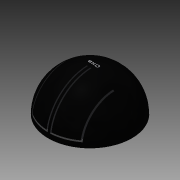
# Autodesk Inventor part: ORB-top
Saved by Autodesk Inventor 2015 (Build 190159000, 159)
## iProperties
Created: 2014-12-21
Part Number: ORB-top
Material: Generic
Document SubType Name: Modeling
Designer: Sudhar
Density: 1 g/cm^3
Appearance: Default
Author: Sudhar
Autodesk Inventor part; units mm, degrees
ref_plane "YZ Plane" through (0, 0, 0) normal (1, 0, 0) x (0, 1, 0)
sketch "Sketch1" plane through (0, 0, 0) normal (0, 0, 1) x (1, 0, 0)
  arc A0 (41.3405, 2.1184) -> (-3.1095, 46.5684) centre (-3.1095, 2.1184) ccw
  line L0 (-3.1095, 46.5684) -> (-3.1095, 2.1184)
  line L1 (41.3405, 2.1184) -> (-3.1095, 2.1184)
  dimension "d0" = 88.9
  constraints: 4 end point, 2 point on circle, 1 centre point, 1 perpendicular, 1 vertical
  measures "d0" diameter of A0
revolve "Revolution1" add sketch "Sketch1" angle 360 about axis through (-3.1095, 46.5684, 0) along (0, -1, 0)
shell "Shell1" thickness 3.175 removed faces 1 at (2.5499, 2.1184, 0)
ref_plane "Work Plane1" through (-3.1095, 2.1184, 44.45) normal (0, 0, 1) x (1, 0, 0)
sketch "Sketch2" plane through (-3.1095, 2.1184, 44.45) normal (0, 0, 1) x (1, 0, 0)
  line L0 (-26.3059, 36.8636) -> (-26.3059, 8.2886)
  line L1 (-23.1309, 5.1136) -> (-0.9059, 5.1136)
  line L2 (-0.9059, 5.1136) -> (-0.9059, 45.5389)
  line L3 (-0.9059, 45.5389) -> (1.6341, 45.5389)
  line L4 (1.6341, 45.5389) -> (1.6341, 5.1136)
  line L5 (1.6341, 5.1136) -> (27.0341, 5.1136)
  line L6 (27.0341, 5.1136) -> (27.0341, 36.8636)
  line L7 (-26.3059, 36.8636) -> (-25.0359, 36.8636)
  line L8 (-25.0359, 36.8636) -> (-25.0359, 9.7512)
  line L9 (-21.8609, 6.5762) -> (-2.1759, 6.5762)
  line L10 (-2.1759, 6.5762) -> (-2.1759, 46.5552)
  line L11 (-2.1759, 46.5552) -> (2.9041, 46.5552)
  line L12 (2.9041, 46.5552) -> (2.9041, 6.5762)
  line L13 (2.9041, 6.5762) -> (25.7641, 6.5762)
  line L14 (25.7641, 6.5762) -> (25.7641, 36.8636)
  line L15 (25.7641, 36.8636) -> (27.0341, 36.8636)
  arc A0 (-26.3059, 8.2886) -> (-23.1309, 5.1136) centre (-23.1309, 8.2886) ccw
  arc A1 (-25.0359, 9.7512) -> (-21.8609, 6.5762) centre (-21.8609, 9.7512) ccw
  point P0 (-26.3059, 5.1136)
  point P1 (-25.0359, 6.5762)
  dimension "d3" = 25.4
  dimension "d4" = 25.4
  dimension "d5" = 2.54
  dimension "d6" = 31.75
  dimension "d7" = 31.75
  dimension "d8" = 1.27
  dimension "d9" = 1.27
  dimension "d10" = 1.27
  dimension "d11" = 1.27
  dimension "d16" = 3.175
  constraints: 32 end point, 9 perpendicular, 9 point on line, 4 point on circle, 4 tangent, 2 centre point, 2 parallel, 1 equal radius, 1 horizontal, 1 vertical
  measures "d3" distance of point (-26.306, 5.114) L1.end
  measures "d4" distance of L4.end L5.end
  measures "d5" distance of L2.end L3.end
  measures "d6" distance of L0.start point (-26.306, 5.114)
  measures "d7" distance of L5.end L6.end
  measures "d8" distance of L0.start L7.end
  measures "d9" horizontal distance of L2.end L10.end
  measures "d10" horizontal distance of L3.end L11.end
  measures "d11" horizontal distance of L5.end L13.end
  measures "d16" radius of A0
extrude "Extrusion1" cut sketch "Sketch2" against normal blind 43.18
ref_plane "Work Plane2" through (-3.1095, 46.5684, 0) normal (0, 1, 0) x (-1, 0, 0)
sketch "Sketch3" plane through (-3.1095, 46.5684, 0) normal (0, 1, 0) x (-1, 0, 0)
  line L0 (-11.0824, -2.3342) -> (10.5197, -2.3342) construction
  line L1 (10.5197, -2.3342) -> (10.5197, -7.7787) construction
  line L2 (10.5197, -7.7787) -> (-11.0824, -7.7787) construction
  line L3 (-11.0824, -7.7787) -> (-11.0824, -2.3342) construction
  spline S0 degree 2 poles (-5.7235, -3.0556) (-5.7235, -2.6408) (-5.426, -2.3342) (-5.0081, -2.3342) knots 0 0 0 1 2 2 2
  line L4 (-5.0081, -2.3342) -> (-2.901, -2.3342)
  spline S1 degree 2 poles (-2.901, -2.3342) (-2.4892, -2.3342) (-2.1916, -2.6378) (-2.1916, -3.0556) knots 0 0 0 1 2 2 2
  line L5 (-2.1916, -3.0556) -> (-2.1916, -4.6607)
  spline S2 degree 2 poles (-2.1916, -4.6607) (-2.1916, -5.0816) (-2.4892, -5.3822) (-2.901, -5.3822) knots 0 0 0 1 2 2 2
  line L6 (-2.901, -5.3822) -> (-5.0081, -5.3822)
  spline S3 degree 2 poles (-5.0081, -5.3822) (-5.426, -5.3822) (-5.7235, -5.0756) (-5.7235, -4.6607) knots 0 0 0 1 2 2 2
  line L7 (-5.7235, -4.6607) -> (-5.7235, -3.0556)
  line L8 (-5.2155, -4.9583) -> (-2.6936, -4.9583)
  line L9 (-2.6936, -4.9583) -> (-2.6936, -2.749)
  line L10 (-2.6936, -2.749) -> (-5.2155, -2.749)
  line L11 (-5.2155, -2.749) -> (-5.2155, -4.9583)
  line L12 (-0.857, -5.3822) -> (-0.857, -2.8812)
  line L13 (-0.857, -2.8812) -> (1.157, -2.8812)
  spline S4 degree 2 poles (1.157, -2.8812) (1.4365, -2.8812) (1.68, -3.1097) (1.68, -3.3652) knots 0 0 0 1 2 2 2
  line L14 (1.68, -3.3652) -> (1.68, -3.9243)
  spline S5 degree 2 poles (1.68, -3.9243) (1.68, -4.1768) (1.4365, -4.4022) (1.157, -4.4022) knots 0 0 0 1 2 2 2
  line L15 (1.157, -4.4022) -> (0.8233, -4.4022)
  line L16 (0.8233, -4.4022) -> (1.9265, -5.3822)
  line L17 (1.9265, -5.3822) -> (1.2953, -5.3822)
  line L18 (1.2953, -5.3822) -> (0.2973, -4.4022)
  line L19 (0.2973, -4.4022) -> (-0.385, -4.4022)
  line L20 (-0.385, -4.4022) -> (-0.385, -5.3822)
  line L21 (-0.385, -5.3822) -> (-0.857, -5.3822)
  line L22 (0.9496, -3.248) -> (-0.385, -3.248)
  line L23 (-0.385, -3.248) -> (-0.385, -4.0535)
  line L24 (-0.385, -4.0535) -> (0.9496, -4.0535)
  spline S6 degree 2 poles (0.9496, -4.0535) (1.1089, -4.0535) (1.2171, -3.9513) (1.2171, -3.801) knots 0 0 0 1 2 2 2
  line L25 (1.2171, -3.801) -> (1.2171, -3.5005)
  spline S7 degree 2 poles (1.2171, -3.5005) (1.2171, -3.3622) (1.1029, -3.248) (0.9496, -3.248) knots 0 0 0 1 2 2 2
  line L26 (2.7592, -5.3822) -> (2.7592, -2.8812)
  line L27 (2.7592, -2.8812) -> (4.8723, -2.8812)
  spline S8 degree 2 poles (4.8723, -2.8812) (5.1609, -2.8812) (5.4194, -3.1157) (5.4194, -3.3712) knots 0 0 0 1 2 2 2
  line L28 (5.4194, -3.3712) -> (5.4194, -3.6598)
  spline S9 degree 2 poles (5.4194, -3.6598) (5.4194, -3.8582) (5.212, -4.0626) (4.9865, -4.0866) knots 0 0 0 1 2 2 2
  spline S10 degree 2 poles (4.9865, -4.0866) (5.206, -4.1107) (5.4374, -4.3601) (5.4374, -4.5706) knots 0 0 0 1 2 2 2
  line L29 (5.4374, -4.5706) -> (5.4374, -4.8922)
  spline S11 degree 2 poles (5.4374, -4.8922) (5.4374, -5.1387) (5.0797, -5.3822) (4.713, -5.3822) knots 0 0 0 1 2 2 2
  line L30 (4.713, -5.3822) -> (2.7592, -5.3822)
  line L31 (3.2311, -4.2549) -> (3.2311, -5.0154)
  line L32 (3.2311, -5.0154) -> (4.6829, -5.0154)
  spline S12 degree 2 poles (4.6829, -5.0154) (4.8453, -5.0154) (4.9685, -4.8922) (4.9685, -4.7329) knots 0 0 0 1 2 2 2
  line L33 (4.9685, -4.7329) -> (4.9685, -4.5375)
  spline S13 degree 2 poles (4.9685, -4.5375) (4.9685, -4.3812) (4.8423, -4.2549) (4.6829, -4.2549) knots 0 0 0 1 2 2 2
  line L34 (4.6829, -4.2549) -> (3.2311, -4.2549)
  line L35 (4.9505, -3.6868) -> (4.9505, -3.4524)
  spline S14 degree 2 poles (4.9505, -3.4524) (4.9505, -3.3381) (4.8362, -3.248) (4.6829, -3.248) knots 0 0 0 1 2 2 2
  line L36 (4.6829, -3.248) -> (3.2311, -3.248)
  line L37 (3.2311, -3.248) -> (3.2311, -3.8882)
  line L38 (3.2311, -3.8882) -> (4.6829, -3.8882)
  spline S15 degree 2 poles (4.6829, -3.8882) (4.8453, -3.8882) (4.9505, -3.801) (4.9505, -3.6868) knots 0 0 0 1 2 2 2
  constraints: 2 other
extrude "Extrusion2" add sketch "Sketch3" against normal blind 0.762
body "Solid1"
